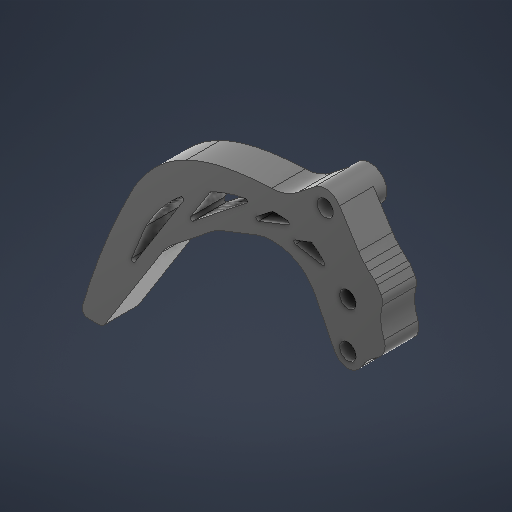
# Autodesk Inventor part: Ring Guide 24
Saved by Autodesk Inventor 2025.1 (Build 291241000, 241)
## iProperties
Created: 2024-12-30
Part Number: Ring Guide 24
Material: Generic
Document SubType Name: Modeling
Designer: Juan
Density: 1 g/cm^3
Appearance: Default
Author: Juan
Autodesk Inventor part; units mm, degrees
ref_plane "YZ Plane" through (0, 0, 0) normal (1, 0, 0) x (0, 1, 0)
ref_plane "XZ Plane" through (0, 0, 0) normal (0, 1, 0) x (-1, 0, 0)
ref_plane "XY Plane" through (0, 0, 0) normal (0, 0, 1) x (1, 0, 0)
sketch "Sketch1" plane through (0, 0, 0) normal (0, 0, 1) x (1, 0, 0)
  circle A0 centre (0, 0) radius 2.3241
  line L0 (0, 0) -> (0, 12.7)
  line L1 (0, 0) -> (0, 6.35)
  line L2 (0, 6.35) -> (6.35, 6.35)
  line L3 (6.35, 6.35) -> (6.35, 19.05)
  circle A1 centre (0, 12.7) radius 2.3241
  circle A2 centre (6.35, 6.35) radius 2.3241
  circle A3 centre (6.35, 19.05) radius 2.3241
  line L4 (0, 0) -> (6.35, 19.05) construction
  line L5 (3.91569, -1.30523) -> (10.26569, 17.74477)
  line L6 (2.43431, 20.35523) -> (-3.91569, 1.30523)
  arc A4 (-3.91569, 1.30523) -> (3.91569, -1.30523) centre (0, 0) ccw
  arc A5 (10.26569, 17.74477) -> (2.43431, 20.35523) centre (6.35, 19.05) ccw
  line L7 (6.35, 6.35) -> (0, 12.7) construction
  line L8 (9.268583, 9.268583) -> (2.918583, 15.618583)
  line L9 (-2.918583, 9.781417) -> (3.431417, 3.431417)
  arc A6 (3.431417, 3.431417) -> (9.268583, 9.268583) centre (6.35, 6.35) ccw
  arc A7 (2.918583, 15.618583) -> (-2.918583, 9.781417) centre (0, 12.7) ccw
  point P0 (3.175, 9.525)
  point P1 (3.175, 9.525)
  point P2 (7.18979, 8.51707)
  point P3 (5.72159, 4.11247)
  point P4 (-0.83979, 10.53293)
  point P5 (0.62841, 14.93753)
  point P6 (7.897367, 10.6398)
  point P7 (1.199064, 16.649494)
  point P8 (-1.547367, 8.4102)
  point P9 (5.150936, 2.400506)
  dimension "d0" = 4.6482
  dimension "d1" = 12.7
  dimension "d2" = 6.35
  dimension "d3" = 12.7
  dimension "d4" = 4.6482
  dimension "d5" = 4.6482
  dimension "d6" = 4.6482
  dimension "d7" = 8.255
  dimension "d8" = 8.255
  constraints: 24 end point, 8 centre point, 8 point on circle, 8 tangent, 4 coincident, 3 midpoint, 2 parallel, 2 perpendicular, 1 vertical
  measures "d0" diameter of A0
  measures "d1" distance of L0.start L0.end
  measures "d2" distance of L1.end L2.end
  measures "d3" distance of L2.end L3.end
  measures "d4" diameter of A1
  measures "d5" diameter of A2
  measures "d6" diameter of A3
  measures "d7" diameter of A5
  measures "d8" diameter of A7
sketch "Sketch1 outline for Extrusion1" plane through (0, 0, 0) normal (0, 0, 1) x (1, 0, 0)
  line L0 (7.897367, 10.6398) -> (10.26569, 17.74477)
  line L1 (9.268583, 9.268583) -> (7.897367, 10.6398)
  arc A0 (10.26569, 17.74477) -> (2.43431, 20.35523) centre (6.35, 19.05) ccw
  arc A1 (5.150936, 2.400506) -> (9.268583, 9.268583) centre (6.35, 6.35) ccw
  line L2 (2.43431, 20.35523) -> (1.199064, 16.649494)
  line L3 (3.91569, -1.30523) -> (5.150936, 2.400506)
  arc A2 (1.199064, 16.649494) -> (-2.918583, 9.781417) centre (0, 12.7) ccw
  arc A3 (-3.91569, 1.30523) -> (3.91569, -1.30523) centre (0, 0) ccw
  line L4 (-2.918583, 9.781417) -> (-1.547367, 8.4102)
  line L5 (-1.547367, 8.4102) -> (-3.91569, 1.30523)
  arc A4 (7.18979, 8.51707) -> (5.72159, 4.11247) centre (6.35, 6.35) cw
  line L6 (5.72159, 4.11247) -> (7.18979, 8.51707)
  arc A5 (-0.83979, 10.53293) -> (0.62841, 14.93753) centre (0, 12.7) cw
  line L7 (0.62841, 14.93753) -> (-0.83979, 10.53293)
extrude "Extrusion1" add sketch "Sketch1 outline for Extrusion1" along normal blind 9.525
sketch "Sketch1 outline for Extrusion2" plane through (0, 0, 0) normal (0, 0, 1) x (1, 0, 0)
  line L0 (0.62841, 14.93753) -> (-0.83979, 10.53293)
  arc A0 (-0.83979, 10.53293) -> (0.62841, 14.93753) centre (0, 12.7) ccw
  circle A1 centre (6.35, 19.05) radius 2.3241
  circle A2 centre (0, 0) radius 2.3241
  line L1 (5.72159, 4.11247) -> (7.18979, 8.51707)
  arc A3 (7.18979, 8.51707) -> (5.72159, 4.11247) centre (6.35, 6.35) ccw
extrude "Extrusion2" cut sketch "Sketch1 outline for Extrusion2" along normal blind 25.4
sketch "Sketch2" plane through (0, 0, 9.525) normal (0, 0, 1) x (1, 0, 0)
  line L0 (12.084555, 18.493301) -> (2.43431, 24.05443)
  line L1 (2.43431, 24.05443) -> (11.536275, 23.23201)
  line L2 (11.536275, 23.23201) -> (12.084555, 18.493301)
  point P0 (0, 0)
  constraints: 6 end point
sketch "Sketch2 outline for Extrusion3" plane through (0, 0, 9.525) normal (0, 0, 1) x (1, 0, 0)
  line L0 (12.084555, 18.493301) -> (11.536275, 23.23201)
  line L1 (2.43431, 24.05443) -> (12.084555, 18.493301)
  line L2 (11.536275, 23.23201) -> (2.43431, 24.05443)
extrude "Extrusion3" cut sketch "Sketch2 outline for Extrusion3" against normal blind 9.525
sketch "Sketch1 outline for Extrusion4" plane through (0, 0, 0) normal (0, 0, 1) x (1, 0, 0)
  circle A0 centre (6.35, 19.05) radius 2.3241
extrude "Extrusion4" add sketch "Sketch1 outline for Extrusion4" along normal blind 12.7
sketch "Sketch3" plane through (0, 0, 9.525) normal (0, 0, 1) x (1, 0, 0)
  line L0 (10.488972, 16.514463) -> (6.256896, 23.507248)
  line L1 (6.256896, 23.507248) -> (14.031842, 17.74477)
  line L2 (14.031842, 17.74477) -> (10.488972, 16.514463)
  point P0 (0, 0)
  constraints: 6 end point
sketch "Sketch3 outline for Extrusion5" plane through (0, 0, 9.525) normal (0, 0, 1) x (1, 0, 0)
  line L0 (10.488972, 16.514463) -> (14.031842, 17.74477)
  line L1 (6.256896, 23.507248) -> (10.488972, 16.514463)
  line L2 (14.031842, 17.74477) -> (6.256896, 23.507248)
extrude "Extrusion5" cut sketch "Sketch3 outline for Extrusion5" against normal through all
fillet "Fillet1" radius 3.175 3 edges at (10.0805, 17.1893, 4.7625) (7.7955, 20.9649, 4.7625) (4.6175, 22.7963, 4.7625)
sketch "Sketch1 outline for Extrusion6" plane through (0, 0, 0) normal (0, 0, 1) x (1, 0, 0)
  circle A0 centre (6.35, 6.35) radius 2.3241
extrude "Extrusion6" add sketch "Sketch1 outline for Extrusion6" along normal blind 12.7
fillet "Fillet2" radius 12.7 4 edges at (7.8974, 10.6398, 4.7625) (5.1509, 2.4005, 4.7625) (-1.5474, 8.4102, 4.7625) (1.1991, 16.6495, 4.7625)
sketch "Sketch5" plane through (0, 0, 9.525) normal (0, 0, 1) x (1, 0, 0)
  circle A0 centre (0, 12.7) radius 2.3241
  circle A1 centre (6.35, 19.05) radius 2.3241
  circle A2 centre (0, 0) radius 2.3241
  circle A3 centre (6.35, 6.35) radius 2.3241
  line L0 (0, 0) -> (0, 12.7)
  line L1 (0, 12.7) -> (0, 28.575)
  line L2 (0, 12.7) -> (-6.253828, 27.291274)
  line L3 (-50.886562, 6.334533) -> (-50.847588, 19.034473)
  ellipse E0 centre (-11.868541, 28.439883) end of major axis (-6.368566, 28.423004) minor radius 0.016782
  arc A4 (-11.868541, 28.439883) -> (-50.840694, 21.280921) centre (-18.848981, -43.21813) ccw
  arc A5 (-50.840694, 21.280921) -> (-82.889743, -76.117644) centre (88.849183, -78.656268) ccw
  arc A6 (-37.882466, 26.217623) -> (-58.057278, 10.333592) centre (-30.14162, -4.368622) ccw
  line L4 (0, 27.13034) -> (-11.1125, 27.13034)
  dimension "d23" = 15.875
  dimension "d24" = 23.2
  dimension "d25" = 15.875
  dimension "d26" = 11.1125
  constraints: 10 end point, 8 point on circle, 4 centre point, 2 point on line, 1 horizontal, 1 vertical
  measures "d23" distance of L0.end L1.end
  measures "d24" angle of L1 L2
  measures "d25" distance of L0.end L2.end
  measures "d26" distance of L4.start L4.end
sketch "Sketch6" plane through (0, 0, 9.525) normal (0, 0, 1) x (1, 0, 0)
  arc A0 (6.836752, 21.517443) -> (2.600408, 20.51364) centre (5.251485, 18.766524) ccw
  line L0 (6.836752, 21.517443) -> (0, 28.544079)
  line L1 (0, 28.544079) -> (-6.396582, 28.544079)
  arc A1 (-50.670577, 21.517443) -> (-60.826209, 8.567162) centre (-22.854372, -10.753246) ccw
  line L2 (-6.396582, 28.544079) -> (-25.868409, 28.544079)
  arc A2 (-25.868409, 28.544079) -> (-50.670577, 21.517443) centre (-20.428097, -37.944649) ccw
  arc A3 (-60.664768, 8.881229) -> (-75.231111, -28.444205) centre (111.460489, -79.796076) ccw
  line L3 (-75.231111, -28.444205) -> (-68.881111, -28.444205)
  arc A4 (-56.817862, 2.110935) -> (-68.881111, -28.444205) centre (954.768206, -414.924778) ccw
  arc A5 (-1.963221, 16.330705) -> (2.600408, 20.51364) centre (-8.0039, 27.502106) ccw
  arc A6 (0, 17.641701) -> (-56.817862, 2.110935) centre (-21.137025, -16.727271) ccw
  point P0 (0, 0)
  dimension "d27" = 6.35
  constraints: 13 point on circle, 8 end point, 5 centre point, 3 horizontal
  measures "d27" distance of L3.start L3.end
sketch "Sketch6 outline for Extrusion7" plane through (0, 0, 9.525) normal (0, 0, 1) x (1, 0, 0)
  arc A0 (-25.868409, 28.544079) -> (-50.670577, 21.517443) centre (-20.428097, -37.944649) ccw
  line L0 (-6.396582, 28.544079) -> (-25.868409, 28.544079)
  line L1 (0, 28.544079) -> (-6.396582, 28.544079)
  line L2 (6.836752, 21.517443) -> (0, 28.544079)
  arc A1 (2.600408, 20.51364) -> (6.836752, 21.517443) centre (5.251485, 18.766524) cw
  arc A2 (0, 17.641701) -> (2.600408, 20.51364) centre (-8.0039, 27.502106) ccw
  arc A3 (-56.817862, 2.110935) -> (0, 17.641701) centre (-21.137025, -16.727271) cw
  arc A4 (-68.881111, -28.444205) -> (-56.817862, 2.110935) centre (954.768206, -414.924778) cw
  line L3 (-75.231111, -28.444205) -> (-68.881111, -28.444205)
  arc A5 (-60.664768, 8.881229) -> (-75.231111, -28.444205) centre (111.460489, -79.796076) ccw
  arc A6 (-50.670577, 21.517443) -> (-60.664768, 8.881229) centre (-22.854372, -10.753246) ccw
extrude "Extrusion7" add sketch "Sketch6 outline for Extrusion7" against normal up to surface (9.525 mm away)
fillet "Fillet3" radius 12.7 4 edges at (0, 28.5441, 4.7625) (-50.6706, 21.5174, 4.7625) (-60.6648, 8.8812, 4.7625) (-25.8684, 28.5441, 4.7625)
fillet "Fillet4" radius 12.7 1 edges at (0, 17.6417, 4.7625)
sketch "Sketch7" plane through (0, 0, 9.525) normal (0, 0, 1) x (1, 0, 0)
  arc A0 (-25.322288, 28.544079) -> (-26.473097, 28.491831) centre (-25.322288, 15.844079) ccw
  arc A1 (-26.473097, 28.491831) -> (-48.900393, 22.385081) centre (-20.428097, -37.944649) ccw
  arc A2 (-48.900393, 22.385081) -> (-52.239444, 20.095679) centre (-43.480019, 10.899893) ccw
  arc A3 (-52.239444, 20.095679) -> (-60.652245, 8.905324) centre (-22.854372, -10.753246) ccw
  arc A4 (-60.652245, 8.905324) -> (-60.675545, 8.860306) centre (-49.385041, 3.045281) ccw
  arc A5 (-60.675545, 8.860306) -> (-75.231111, -28.444205) centre (111.460489, -79.796076) ccw
  line L0 (-75.231111, -28.444205) -> (-68.881111, -28.444205)
  arc A6 (-56.817862, 2.110935) -> (-68.881111, -28.444205) centre (954.768206, -414.924778) ccw
  arc A7 (-14.648845, 23.096134) -> (-56.817862, 2.110935) centre (-21.137025, -16.727271) ccw
  arc A8 (-4.094031, 12.175439) -> (-14.648845, 23.096134) centre (-16.691051, 10.561407) ccw
  arc A9 (-4.094031, 12.175439) -> (-3.827415, 11.15496) centre (0, 12.7) ccw
  arc A10 (-3.5558, 2.3849) -> (-3.827415, 11.15496) centre (-15.604078, 6.400992) ccw
  line L1 (-3.5558, 2.3849) -> (-3.91569, 1.30523)
  arc A11 (-3.91569, 1.30523) -> (3.591537, -2.03399) centre (0, 0) ccw
  arc A12 (8.38399, 2.758463) -> (3.591537, -2.03399) centre (14.642421, -8.292421) ccw
  arc A13 (8.38399, 2.758463) -> (10.173394, 7.904964) centre (6.35, 6.35) ccw
  arc A14 (9.671027, 15.978707) -> (10.173394, 7.904964) centre (21.937685, 12.689467) ccw
  arc A15 (9.671027, 15.978707) -> (9.320644, 18.444927) centre (6.604362, 16.801017) ccw
  line L2 (9.320644, 18.444927) -> (8.598411, 19.638294)
  arc A16 (7.583467, 21.019772) -> (8.598411, 19.638294) centre (6.35, 19.05) ccw
  arc A17 (7.583467, 21.019772) -> (7.087567, 21.372906) centre (5.5023, 18.621987) ccw
  line L3 (7.087567, 21.372906) -> (6.836752, 21.517443)
  line L4 (6.836752, 21.517443) -> (3.739709, 24.700503)
  arc A18 (3.739709, 24.700503) -> (-5.362695, 28.544079) centre (-5.362695, 15.844079) ccw
  line L5 (-5.362695, 28.544079) -> (-25.322288, 28.544079)
  circle A19 centre (6.35, 6.35) radius 2.3241
  circle A20 centre (0, 0) radius 2.3241
  circle A21 centre (0, 12.7) radius 2.3241
  line L6 (-68.881111, -28.444205) -> (-38.616893, 19.638294)
  line L7 (-50.977682, 0) -> (-21.137025, 23.621212)
  line L8 (-36.88563, 11.15496) -> (-10.268024, 21.517443)
  line L9 (-22.382878, 16.801017) -> (-4.384406, 13.697725)
  line L10 (-12.077114, 15.0241) -> (-3.696088, -1.837169)
  line L11 (-68.881111, -28.444205) -> (-71.20998, -26.183883)
  line L12 (-38.616893, 19.638294) -> (-41.300871, 21.334433)
  line L13 (-41.300871, 21.334433) -> (-71.20998, -26.183883)
  line L14 (-50.977682, 0) -> (-52.948278, 2.489453)
  line L15 (-52.948278, 2.489453) -> (-26.747773, 23.2292)
  line L16 (-36.88563, 11.15496) -> (-38.037478, 14.113655)
  line L17 (-38.037478, 14.113655) -> (-14.872624, 23.131948)
  line L18 (-22.382878, 16.801017) -> (-21.843406, 19.92985)
  line L19 (-21.843406, 19.92985) -> (-5.847007, 17.171755)
  line L20 (-12.077114, 15.0241) -> (-9.23397, 16.437307)
  line L21 (-9.23397, 16.437307) -> (-3.110855, 4.11859)
  point P0 (-45.898104, 8.070217)
  point P1 (-44.594351, 16.101892)
  point P2 (-62.923811, -13.019172)
  point P3 (-16.647287, 19.033936)
  point P4 (-28.415873, 17.859435)
  dimension "d32" = 3.175
  dimension "d33" = 3.175
  dimension "d34" = 3.175
  dimension "d35" = 3.175
  dimension "d36" = 3.175
  constraints: 32 end point, 9 point on circle, 8 perpendicular, 4 point on line, 1 parallel, 1 tangent
  measures "d32" distance of L6.end L12.end
  measures "d33" distance of L7.start L14.end
  measures "d34" distance of L8.start L16.end
  measures "d35" distance of L9.start L18.end
  measures "d36" distance of L10.start L20.end
sketch "Sketch7 outline for Extrusion8" plane through (0, 0, 9.525) normal (0, 0, 1) x (1, 0, 0)
  line L0 (-45.898104, 8.070217) -> (-38.616893, 19.638294)
  line L1 (-26.747773, 23.2292) -> (-45.898104, 8.070217)
  arc A0 (-21.137025, 23.621212) -> (-26.747773, 23.2292) centre (-21.137025, -16.727271) ccw
  line L2 (-28.415873, 17.859435) -> (-21.137025, 23.621212)
  line L3 (-14.872624, 23.131948) -> (-28.415873, 17.859435)
  arc A1 (-14.648845, 23.096134) -> (-14.872624, 23.131948) centre (-21.137025, -16.727271) ccw
  arc A2 (-10.268024, 21.517443) -> (-14.648845, 23.096134) centre (-16.691051, 10.561407) ccw
  line L4 (-16.647287, 19.033936) -> (-10.268024, 21.517443)
  line L5 (-5.847007, 17.171755) -> (-16.647287, 19.033936)
  arc A3 (-4.094031, 12.175439) -> (-5.847007, 17.171755) centre (-16.691051, 10.561407) ccw
  arc A4 (-3.827415, 11.15496) -> (-4.094031, 12.175439) centre (0, 12.7) cw
  arc A5 (-3.5558, 2.3849) -> (-3.827415, 11.15496) centre (-15.604078, 6.400992) ccw
  line L6 (-3.91569, 1.30523) -> (-3.5558, 2.3849)
  arc A6 (-3.696088, -1.837169) -> (-3.91569, 1.30523) centre (0, 0) cw
  line L7 (-12.077114, 15.0241) -> (-3.696088, -1.837169)
  line L8 (-22.382878, 16.801017) -> (-12.077114, 15.0241)
  line L9 (-36.88563, 11.15496) -> (-22.382878, 16.801017)
  line L10 (-50.977682, 0) -> (-36.88563, 11.15496)
  line L11 (-68.881111, -28.444205) -> (-50.977682, 0)
  arc A7 (-62.923811, -13.019172) -> (-68.881111, -28.444205) centre (954.768206, -414.924778) ccw
  line L12 (-44.594351, 16.101892) -> (-62.923811, -13.019172)
  arc A8 (-38.616893, 19.638294) -> (-44.594351, 16.101892) centre (-21.137025, -16.727271) ccw
extrude "Extrusion8" add sketch "Sketch7 outline for Extrusion8" against normal up to surface (9.525 mm away)
fillet "Fillet5" radius 0.529167 9 edges at (-44.5944, 16.1019, 4.7625) (-62.9238, -13.0192, 4.7625) (-45.8981, 8.0702, 4.7625) (-26.7478, 23.2292, 4.7625) (-28.4159, 17.8594, 4.7625) (-14.8726, 23.1319, 4.7625) (-16.6473, 19.0339, 4.7625) (-5.847, 17.1718, 4.7625) (-10.268, 21.5174, 4.7625)
fillet "Fillet6" radius 1.5875 2 edges at (-38.6169, 19.6383, 4.7625) (-21.137, 23.6212, 4.7625)
fillet "Fillet7" radius 1.5875 2 edges at (-75.2311, -28.4442, 4.7625) (-68.8811, -28.4442, 4.7625)
fillet "Fillet8" radius 12.7 4 edges at (-50.9777, 0, 4.7625) (-36.8856, 11.155, 4.7625) (-22.3829, 16.801, 4.7625) (-12.0771, 15.0241, 4.7625)
sketch "Sketch8" plane through (0, 0, 9.525) normal (0, 0, 1) x (1, 0, 0)
  arc A0 (-6.563353, 18.224288) -> (-10.040765, 21.381005) centre (-16.691051, 10.561407) ccw
  arc A1 (-7.075253, 17.383529) -> (-6.563353, 18.224288) centre (-6.985341, 17.905001) ccw
  line L0 (-7.075253, 17.383529) -> (-14.770365, 18.710318)
  arc A2 (-14.872427, 19.724906) -> (-14.770365, 18.710318) centre (-14.680452, 19.23179) ccw
  line L1 (-14.872427, 19.724906) -> (-10.509835, 21.423304)
  arc A3 (-10.040765, 21.381005) -> (-10.509835, 21.423304) centre (-10.31786, 20.930188) ccw
  line L2 (-16.797983, 22.382388) -> (-25.134566, 19.136879)
  arc A4 (-25.654973, 20.044903) -> (-25.134566, 19.136879) centre (-25.32654, 19.629994) ccw
  line L3 (-25.654973, 20.044903) -> (-21.574934, 23.274573)
  arc A5 (-20.567217, 23.617188) -> (-21.574934, 23.274573) centre (-20.589636, 22.029847) ccw
  arc A6 (-16.934846, 23.401793) -> (-20.567217, 23.617188) centre (-21.137025, -16.727271) ccw
  arc A7 (-16.797983, 22.382388) -> (-16.934846, 23.401793) centre (-16.989957, 22.875504) ccw
  line L4 (-28.357406, 21.95505) -> (-43.476944, 9.986754)
  arc A8 (-44.253217, 10.683544) -> (-43.476944, 9.986754) centre (-43.805377, 10.401663) ccw
  line L5 (-44.253217, 10.683544) -> (-38.863152, 19.247049)
  arc A9 (-38.1906, 19.840142) -> (-38.863152, 19.247049) centre (-37.519632, 18.401407) ccw
  arc A10 (-28.786157, 22.889529) -> (-38.1906, 19.840142) centre (-21.137025, -16.727271) ccw
  arc A11 (-28.357406, 21.95505) -> (-28.786157, 22.889529) centre (-28.685839, 22.369959) ccw
  line L6 (-46.181383, 13.580484) -> (-59.852083, -8.138942)
  arc A12 (-60.791068, -7.660099) -> (-59.852083, -8.138942) centre (-60.299923, -7.857061) ccw
  arc A13 (-56.817862, 2.110935) -> (-60.791068, -7.660099) centre (954.768206, -414.924778) ccw
  arc A14 (-46.967993, 14.268877) -> (-56.817862, 2.110935) centre (-21.137025, -16.727271) ccw
  arc A15 (-46.181383, 13.580484) -> (-46.967993, 14.268877) centre (-46.629223, 13.862365) ccw
  arc A16 (-69.757689, -28.444205) -> (-68.414169, -27.702347) centre (-69.757689, -26.856705) ccw
  line L7 (-68.414169, -27.702347) -> (-52.137008, -1.841888)
  arc A17 (-49.271234, 1.350787) -> (-52.137008, -1.841888) centre (-41.388849, -8.607024) ccw
  line L8 (-49.271234, 1.350787) -> (-38.382093, 9.970393)
  arc A18 (-35.107097, 11.84736) -> (-38.382093, 9.970393) centre (-30.499707, 0.012582) ccw
  line L9 (-35.107097, 11.84736) -> (-25.670978, 15.520929)
  arc A19 (-18.905698, 16.201483) -> (-25.670978, 15.520929) centre (-21.063588, 3.686152) ccw
  line L10 (-18.905698, 16.201483) -> (-18.42475, 16.118558)
  arc A20 (-9.210062, 9.256056) -> (-18.42475, 16.118558) centre (-20.58264, 3.603227) ccw
  line L11 (-9.210062, 9.256056) -> (-3.696088, -1.837169)
  arc A21 (-3.696088, -1.837169) -> (3.591537, -2.03399) centre (0, 0) ccw
  arc A22 (8.38399, 2.758463) -> (3.591537, -2.03399) centre (14.642421, -8.292421) ccw
  arc A23 (8.38399, 2.758463) -> (10.173394, 7.904964) centre (6.35, 6.35) ccw
  arc A24 (9.671027, 15.978707) -> (10.173394, 7.904964) centre (21.937685, 12.689467) ccw
  arc A25 (9.671027, 15.978707) -> (9.320644, 18.444927) centre (6.604362, 16.801017) ccw
  line L12 (9.320644, 18.444927) -> (8.598411, 19.638294)
  arc A26 (7.583467, 21.019772) -> (8.598411, 19.638294) centre (6.35, 19.05) ccw
  arc A27 (7.583467, 21.019772) -> (7.087567, 21.372906) centre (5.5023, 18.621987) ccw
  line L13 (7.087567, 21.372906) -> (6.836752, 21.517443)
  line L14 (6.836752, 21.517443) -> (3.739709, 24.700503)
  arc A28 (3.739709, 24.700503) -> (-5.362695, 28.544079) centre (-5.362695, 15.844079) ccw
  line L15 (-5.362695, 28.544079) -> (-25.322288, 28.544079)
  arc A29 (-25.322288, 28.544079) -> (-26.473097, 28.491831) centre (-25.322288, 15.844079) ccw
  arc A30 (-26.473097, 28.491831) -> (-48.900393, 22.385081) centre (-20.428097, -37.944649) ccw
  arc A31 (-48.900393, 22.385081) -> (-52.239444, 20.095679) centre (-43.480019, 10.899893) ccw
  arc A32 (-52.239444, 20.095679) -> (-60.652245, 8.905324) centre (-22.854372, -10.753246) ccw
  arc A33 (-60.652245, 8.905324) -> (-60.675545, 8.860306) centre (-49.385041, 3.045281) ccw
  arc A34 (-60.675545, 8.860306) -> (-74.662224, -26.419076) centre (111.460489, -79.796076) ccw
  arc A35 (-74.662224, -26.419076) -> (-73.136236, -28.444205) centre (-73.136236, -26.856705) ccw
  line L16 (-73.136236, -28.444205) -> (-69.757689, -28.444205)
  circle A36 centre (6.35, 6.35) radius 2.3241
  circle A37 centre (0, 0) radius 2.3241
  circle A38 centre (0, 12.7) radius 2.3241
  spline S0 degree 4 poles (-74.662224, -26.419076) (-51.589622, 31.8918) (-69.889434, 47.245862) (91.217289, 8.612587) (-63.341829, 41.230273) knots 0 0 0 0 0 1 1 1 1 1
  line L17 (-82.490449, -46.203176) -> (-66.833999, -6.634977) construction
  arc A39 (-81.487834, -41.974225) -> (-68.99644, -10.405004) centre (-289.772202, 58.696211) ccw construction
  point P0 (-45.427874, 23.904838)
  point P1 (-59.685147, 10.662464)
  constraints: 2 end point, 2 midpoint, 2 point on circle, 1 centre point, 6 other
sketch "Sketch8 outline for Extrusion9" plane through (0, 0, 9.525) normal (0, 0, 1) x (1, 0, 0)
  arc A0 (-48.900393, 22.385081) -> (-52.239444, 20.095679) centre (-43.480019, 10.899893) ccw
  arc A1 (-45.427874, 23.904838) -> (-48.900393, 22.385081) centre (-20.428097, -37.944649) ccw
  spline S0 degree 4 poles (-59.685147, 10.662464) (-56.872597, 15.219478) (-53.653756, 18.900684) (-49.807306, 21.758338) (-45.427874, 23.904838) knots 0 0 0 0 0 1 1 1 1 1
  arc A2 (-52.239444, 20.095679) -> (-59.685147, 10.662464) centre (-22.854372, -10.753246) ccw
extrude "Extrusion9" cut sketch "Sketch8 outline for Extrusion9" against normal through all
sketch "Sketch8 outline for Extrusion10" plane through (0, 0, 9.525) normal (0, 0, 1) x (1, 0, 0)
  arc A0 (-26.473097, 28.491831) -> (-25.322288, 28.544079) centre (-25.322288, 15.844079) cw
  arc A1 (-45.427874, 23.904838) -> (-26.473097, 28.491831) centre (-20.428097, -37.944649) cw
  spline S0 degree 4 poles (-45.427874, 23.904838) (-36.578354, 28.242273) (-25.552544, 29.675903) (-13.131195, 29.133126) (-5.362695, 28.544079) knots 0 0 0 0 0 1 1 1 1 1
  line L0 (-25.322288, 28.544079) -> (-5.362695, 28.544079)
extrude "Extrusion10" add sketch "Sketch8 outline for Extrusion10" against normal up to surface (9.525 mm away)
sketch "Sketch9" plane through (0, 0, 9.525) normal (0, 0, 1) x (1, 0, 0)
  circle A0 centre (6.277981, 12.702375) radius 14.66569
  point P0 (0, 0)
  constraints: 1 centre point
sketch "Sketch9 outline for Extrusion11" plane through (0, 0, 9.525) normal (0, 0, 1) x (1, 0, 0)
  circle A0 centre (6.277981, 12.702375) radius 14.66569
extrude "Extrusion11" cut sketch "Sketch9 outline for Extrusion11" along normal blind 25.4
sketch "Sketch10" plane through (0, 0, 0) normal (0, 0, -1) x (-1, 0, 0)
  circle A0 centre (0, 12.7) radius 2.3241
  circle A1 centre (0, 12.7) radius 2.3241
  circle A2 centre (0, 0) radius 2.3241
  line L0 (10.509835, 21.423304) -> (14.872427, 19.724906)
  arc A3 (14.770365, 18.710318) -> (14.872427, 19.724906) centre (14.680452, 19.23179) ccw
  line L1 (14.770365, 18.710318) -> (7.075253, 17.383529)
  arc A4 (6.563353, 18.224288) -> (7.075253, 17.383529) centre (6.985341, 17.905001) ccw
  arc A5 (10.040765, 21.381005) -> (6.563353, 18.224288) centre (16.691051, 10.561407) ccw
  arc A6 (10.509835, 21.423304) -> (10.040765, 21.381005) centre (10.31786, 20.930188) ccw
  arc A7 (56.817862, 2.110935) -> (46.967993, 14.268877) centre (21.137025, -16.727271) ccw
  arc A8 (60.791068, -7.660099) -> (56.817862, 2.110935) centre (-954.768206, -414.924778) ccw
  arc A9 (59.852083, -8.138942) -> (60.791068, -7.660099) centre (60.299923, -7.857061) ccw
  line L2 (59.852083, -8.138942) -> (46.181383, 13.580484)
  arc A10 (46.967993, 14.268877) -> (46.181383, 13.580484) centre (46.629223, 13.862365) ccw
  arc A11 (38.1906, 19.840142) -> (28.786157, 22.889529) centre (21.137025, -16.727271) ccw
  arc A12 (38.863152, 19.247049) -> (38.1906, 19.840142) centre (37.519632, 18.401407) ccw
  line L3 (38.863152, 19.247049) -> (44.253217, 10.683544)
  arc A13 (43.476944, 9.986754) -> (44.253217, 10.683544) centre (43.805377, 10.401663) ccw
  line L4 (43.476944, 9.986754) -> (28.357406, 21.95505)
  arc A14 (28.786157, 22.889529) -> (28.357406, 21.95505) centre (28.685839, 22.369959) ccw
  arc A15 (20.567217, 23.617188) -> (16.934846, 23.401793) centre (21.137025, -16.727271) ccw
  arc A16 (21.574934, 23.274573) -> (20.567217, 23.617188) centre (20.589636, 22.029847) ccw
  line L5 (21.574934, 23.274573) -> (25.654973, 20.044903)
  arc A17 (25.134566, 19.136879) -> (25.654973, 20.044903) centre (25.32654, 19.629994) ccw
  line L6 (25.134566, 19.136879) -> (16.797983, 22.382388)
  arc A18 (16.934846, 23.401793) -> (16.797983, 22.382388) centre (16.989957, 22.875504) ccw
  spline S0 degree 4 poles (45.427874, 23.904838) (36.578354, 28.242273) (25.552544, 29.675903) (13.131195, 29.133126) (5.362695, 28.544079) knots 0 0 0 0 0 1 1 1 1 1
  arc A19 (5.362695, 28.544079) -> (-3.739709, 24.700503) centre (5.362695, 15.844079) ccw
  line L7 (-3.739709, 24.700503) -> (-6.836752, 21.517443)
  line L8 (-6.836752, 21.517443) -> (-7.087567, 21.372906)
  arc A20 (-7.087567, 21.372906) -> (-8.218581, 20.265897) centre (-5.5023, 18.621987) ccw
  line L9 (-8.218581, 20.265897) -> (-9.320644, 18.444927)
  arc A21 (-9.320644, 18.444927) -> (-9.671027, 15.978707) centre (-6.604362, 16.801017) ccw
  arc A22 (-10.173394, 7.904964) -> (-9.671027, 15.978707) centre (-21.937685, 12.689467) ccw
  arc A23 (-10.173394, 7.904964) -> (-8.38399, 2.758463) centre (-6.35, 6.35) ccw
  arc A24 (-3.591537, -2.03399) -> (-8.38399, 2.758463) centre (-14.642421, -8.292421) ccw
  arc A25 (-3.591537, -2.03399) -> (3.696088, -1.837169) centre (0, 0) ccw
  line L10 (3.696088, -1.837169) -> (9.210062, 9.256056)
  arc A26 (18.42475, 16.118558) -> (9.210062, 9.256056) centre (20.58264, 3.603227) ccw
  line L11 (18.42475, 16.118558) -> (18.905698, 16.201483)
  arc A27 (25.670978, 15.520929) -> (18.905698, 16.201483) centre (21.063588, 3.686152) ccw
  line L12 (25.670978, 15.520929) -> (35.107097, 11.84736)
  arc A28 (38.382093, 9.970393) -> (35.107097, 11.84736) centre (30.499707, 0.012582) ccw
  line L13 (38.382093, 9.970393) -> (49.271234, 1.350787)
  arc A29 (52.137008, -1.841888) -> (49.271234, 1.350787) centre (41.388849, -8.607024) ccw
  line L14 (52.137008, -1.841888) -> (68.414169, -27.702347)
  arc A30 (68.414169, -27.702347) -> (69.757689, -28.444205) centre (69.757689, -26.856705) ccw
  line L15 (69.757689, -28.444205) -> (73.136236, -28.444205)
  arc A31 (73.136236, -28.444205) -> (74.662224, -26.419076) centre (73.136236, -26.856705) ccw
  arc A32 (74.662224, -26.419076) -> (60.675545, 8.860306) centre (-111.460489, -79.796076) ccw
  arc A33 (60.675545, 8.860306) -> (60.652245, 8.905324) centre (49.385041, 3.045281) ccw
  arc A34 (60.652245, 8.905324) -> (59.685147, 10.662464) centre (22.854372, -10.753246) ccw
  line L16 (0, 0) -> (0, 12.7)
  line L17 (0, 12.7) -> (0, 31.75)
  line L18 (0, 31.75) -> (6.35, 31.75)
  circle A35 centre (6.35, 31.75) radius 2.3241
  circle A36 centre (6.35, 31.75) radius 4.7625
  line L19 (17.407143, 29.027186) -> (9.318386, 35.474257)
  line L20 (-3.739709, 24.700503) -> (2.324223, 34.294509)
  point P0 (1.5875, 31.75)
  point P1 (0.715955, 31.75)
  point P2 (3.036448, 28.329213)
  point P3 (10.123242, 28.844136)
  dimension "d49" = 19.05
  dimension "d50" = 6.35
  dimension "d51" = 4.6482
  dimension "d52" = 9.525
  constraints: 10 end point, 2 centre point, 2 coincident, 2 point on circle, 2 tangent, 2 vertical, 1 perpendicular, 3 other
  measures "d49" distance of L16.end L17.end
  measures "d50" distance of L17.end L18.end
  measures "d51" diameter of A35
  measures "d52" diameter of A36
sketch "Sketch10 outline for Extrusion12" plane through (0, 0, 0) normal (0, 0, -1) x (-1, 0, 0)
  arc A0 (9.318386, 35.474257) -> (2.324223, 34.294509) centre (6.35, 31.75) ccw
  line L0 (2.324223, 34.294509) -> (-3.739709, 24.700503)
  arc A1 (-3.739709, 24.700503) -> (3.036448, 28.329213) centre (5.362695, 15.844079) cw
  arc A2 (3.036448, 28.329213) -> (10.123242, 28.844136) centre (6.35, 31.75) ccw
  spline S0 degree 4 poles (17.407143, 29.027186) (15.493196, 29.02968) (13.622891, 28.99341) (11.82231, 28.927994) (10.123242, 28.844136) knots 0 0 0 0 0 1 1 1 1 1
  line L1 (17.407143, 29.027186) -> (9.318386, 35.474257)
extrude "Extrusion12" add sketch "Sketch10 outline for Extrusion12" against normal up to surface (9.525 mm away)
sketch "Sketch10 outline for Extrusion13" plane through (0, 0, 0) normal (0, 0, -1) x (-1, 0, 0)
  circle A0 centre (6.35, 31.75) radius 2.3241
extrude "Extrusion13" cut sketch "Sketch10 outline for Extrusion13" against normal through all
fillet "Fillet9" radius 12.7 1 edges at (-17.4071, 29.0272, 4.7625)
fillet "Fillet10" radius 12.7 2 edges at (3.7397, 24.7005, 4.7625) (6.8368, 21.5174, 4.7625)
sketch "Sketch11" plane through (0, 0, 0) normal (0, 0, -1) x (-1, 0, 0)
  circle A0 centre (6.35, 31.75) radius 2.3241 projected
  circle A1 centre (6.35, 31.75) radius 4.7625
  point P0 (0, 0)
  dimension "d59" = 9.525
  constraints: 1 centre point, 1 coincident
  measures "d59" diameter of A1
sketch "Sketch11 outline for Extrusion14" plane through (0, 0, 0) normal (0, 0, -1) x (-1, 0, 0)
  circle A0 centre (6.35, 31.75) radius 4.7625
  circle A1 centre (6.35, 31.75) radius 2.3241
extrude "Extrusion14" add sketch "Sketch11 outline for Extrusion14" along normal blind 3.0734
body "Solid1"
